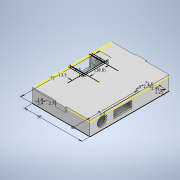
# Autodesk Inventor part: carcasaDisplayAdapter
Saved by Autodesk Inventor 2020 (Build 240168000, 168)
## iProperties
Created: 2021-04-22
Part Number: carcasaDisplayAdapter
Material: Generic
Document SubType Name: Modeling
Designer: Vlasciar
Density: 1 g/cm^3
Appearance: Default
Author: Vlasciar
Autodesk Inventor part; units mm, degrees
ref_plane "YZ Plane" through (0, 0, 0) normal (1, 0, 0) x (0, 1, 0)
ref_plane "XZ Plane" through (0, 0, 0) normal (0, 1, 0) x (-1, 0, 0)
ref_plane "XY Plane" through (0, 0, 0) normal (0, 0, 1) x (1, 0, 0)
sketch "Sketch1" plane through (0, 0, 0) normal (0, 1, 0) x (-1, 0, 0)
  line L0 (-28, -38.5) -> (28, -38.5)
  line L1 (28, -38.5) -> (28, 38.5)
  line L2 (28, 38.5) -> (-28, 38.5)
  line L3 (-28, 38.5) -> (-28, -38.5)
  line L4 (-28, -38.5) -> (28, 38.5) construction
  line L5 (28, -38.5) -> (-28, 38.5) construction
  point P0 (0, 0)
  dimension "d0" = 56
  dimension "d1" = 77
  constraints: 12 end point, 2 midpoint, 2 parallel, 1 horizontal, 1 perpendicular
  measures "d0" distance of L1.end L2.end
  measures "d1" distance of L0.end L1.end
extrude "Extrusion1" add sketch "Sketch1" along normal blind 12.5
shell "Shell1" thickness 1.5 removed faces 1 at (9.3333, 12.5, 12.8333)
sketch "Sketch2" plane through (28, 0, 38.5) normal (1, 0, 0) x (0, 0, -1)
  line L0 (0, 0) -> (77, 0) projected
  line L1 (0, 12.5) -> (77, 12.5) projected
  line L2 (14.3284, 3.5) -> (18, 3.5)
  circle A0 centre (11.5, 7) radius 4.5
  line L3 (1.5, 1.5) -> (1.5, 12.5) projected
  line L4 (40.75, 3.5) -> (23.25, 3.5)
  line L5 (23.25, 3.5) -> (23.25, 10.5)
  line L6 (23.25, 10.5) -> (40.75, 10.5)
  line L7 (40.75, 10.5) -> (40.75, 3.5)
  line L8 (40.75, 3.5) -> (23.25, 10.5) construction
  line L9 (23.25, 3.5) -> (40.75, 10.5) construction
  point P0 (38.5, 0)
  point P1 (32, 7)
  point P2 (32, 7)
  dimension "d10" = 9
  dimension "d7" = 3.5
  dimension "d8" = 3.5
  dimension "d9" = 5.5
  dimension "d11" = 5.5
  dimension "d12" = 17.5
  dimension "d13" = 7
  dimension "d14" = 21.75
  constraints: 14 end point, 3 midpoint, 2 horizontal, 2 parallel, 1 coincident, 1 horizontal alignment, 1 perpendicular, 3 other
  measures "d7" distance between parallel lines of L0 L2
  measures "d8" distance from line of L2 point (11.5, 7)
  measures "d9" distance from line of L1 point (11.5, 7)
  measures "d12" distance of L5.end L6.end
  measures "d13" distance of L6.end L4.start
  measures "d14" distance between parallel lines of L3 L5
extrude "Extrusion2" cut sketch "Sketch2" against normal blind 12.5
sketch "Sketch3" plane through (-28, 0, -38.5) normal (-1, 0, 0) x (0, 0, 1)
  line L0 (0, 0) -> (77, 0) projected
  line L1 (41.3, 3.5) -> (20.5, 3.5)
  line L2 (20.5, 3.5) -> (20.5, 6)
  line L3 (20.5, 6) -> (41.3, 6)
  line L4 (41.3, 6) -> (41.3, 3.5)
  line L5 (41.3, 3.5) -> (20.5, 6) construction
  line L6 (20.5, 3.5) -> (41.3, 6) construction
  line L7 (1.5, 1.5) -> (1.5, 12.5) projected
  line L8 (21.5, 6) -> (21.5, 3.5)
  line L9 (40.3, 6) -> (40.3, 3.4503)
  line L10 (0, 12.5) -> (77, 12.5) projected
  line L11 (21.5, 6) -> (21.5, 12.5)
  line L12 (1.5, 12.5) -> (75.5, 12.5) projected
  line L13 (40.3, 6) -> (40.3, 12.5)
  point P0 (38.5, 0)
  point P1 (30.9, 4.75)
  point P2 (40.3, 3.5)
  dimension "d17" = 3.5
  dimension "d18" = 2.5
  dimension "d19" = 20.8
  dimension "d20" = 19
  dimension "d21" = 1
  dimension "d22" = 1
  constraints: 20 end point, 4 point on line, 3 perpendicular, 2 midpoint, 2 parallel, 2 vertical, 1 horizontal
  measures "d17" distance between parallel lines of L0 L1
  measures "d18" distance of L3.end L1.start
  measures "d19" distance of L2.end L3.end
  measures "d20" distance between parallel lines of L7 L2
  measures "d21" distance between parallel lines of L8 L2
  measures "d22" distance between parallel lines of L4 L9
extrude "Extrusion3" cut sketch "Sketch3" against normal blind 12.5 contours L8 L3 L9 L1
sketch "Sketch4" plane through (-26.5, 1.5, -37) normal (0, 1, 0) x (1, 0, 0)
  line L0 (53, -74) -> (53, 0) projected
  line L1 (53, 0) -> (0, 0) projected
  line L2 (0, 0) -> (0, -74) projected
  line L3 (0, -74) -> (53, -74) projected
  circle A0 centre (3.175, -70.225) radius 1.375
  circle A1 centre (49.375, -3.825) radius 1.375
  point P0 (26.5, -37)
  dimension "d25" = 2.75
  dimension "d26" = 1.8
  dimension "d27" = 2.4
  dimension "d28" = 2.75
  dimension "d29" = 2.25
  dimension "d30" = 2.45
  constraints: 2 centre point
  measures "d25" diameter of A0
  measures "d26" distance edge to line of A0 L2
  measures "d27" distance edge to line of A0 L3
  measures "d28" diameter of A1
  measures "d29" distance edge to line of A1 L0
  measures "d30" distance edge to line of A1 L1
extrude "Extrusion4" add sketch "Sketch4" along normal blind 11 contours A0 | A1
extrude "Extrusion5" cut sketch "Sketch3" against normal blind 10 contours L11 L10 L13 L3
sketch "Sketch5" plane through (0, 12.5, 0) normal (0, 1, 0) x (1, 0, 0)
  line L0 (-28, -1.8) -> (-28, -38.5) projected
  line L1 (-28, -38.5) -> (28, -38.5) projected
  line L2 (28, -38.5) -> (28, 38.5) projected
  line L3 (28, 38.5) -> (-28, 38.5) projected
  line L4 (-28, 38.5) -> (-28, 17) projected
  line L5 (28, 38.5) -> (-28, 38.5) projected
  line L6 (28, 38.5) -> (-28, 38.5)
  line L7 (-28, 38.5) -> (-28, -38.5)
  line L8 (-28, -38.5) -> (28, -38.5)
  line L9 (28, -38.5) -> (28, 38.5)
  point P0 (0, 0)
  constraints: 8 end point, 2 parallel, 1 horizontal, 1 perpendicular
extrude "Extrusion6" add sketch "Sketch5" along normal blind 1.25 separate body
sketch "Sketch6" plane through (0, 13.75, 0) normal (0, 1, 0) x (1, 0, 0)
  line L0 (-28, 38.5) -> (-28, -38.5) projected
  line L1 (-26.5, -1.8) -> (-28, -1.8) projected
  line L2 (-28, -1.8) -> (0, -1.8)
  line L3 (-28, 17) -> (-28, -1.8) projected
  line L4 (-28, 17) -> (0, 17)
  line L5 (-14.5, 22) -> (-14.5, -18)
  line L6 (-14.5, -2.3) -> (-28, -2.3)
  line L7 (-28, 38.5) -> (-28, -38.5) projected
  line L8 (-14.5, 17.5) -> (-28, 17.5)
  line L9 (-14.5, -3.8) -> (-28, -3.8)
  line L10 (-14.5, 19) -> (-28, 19)
  line L11 (-14.5, 19) -> (-13, 19)
  line L12 (-13, 19) -> (-13, -3.8)
  line L13 (-13, -3.8) -> (-14.5, -3.8)
  line L14 (-14.5, -3.8) -> (-14.5, 19)
  line L15 (-26.5, 19) -> (-26.5, 17.5)
  line L16 (-26.5, 37) -> (-26.5, -37) projected
  line L17 (-26.5, -2.3) -> (-26.5, -3.8)
  point P0 (0, 0)
  point P1 (-26.5, -3.8)
  point P2 (-26.5, -2.3)
  dimension "d37" = 13.5
  dimension "d38" = 0.5
  dimension "d39" = 0.5
  dimension "d40" = 1.5
  dimension "d41" = 1.5
  dimension "d42" = 1.5
  dimension "d43" = 18.8
  constraints: 26 end point, 15 point on line, 6 perpendicular, 3 horizontal, 2 parallel, 1 horizontal alignment
  measures "d37" distance between parallel lines of L0 L5
  measures "d38" distance between parallel lines of L2 L6
  measures "d39" distance between parallel lines of L4 L8
  measures "d40" distance between parallel lines of L8 L10
  measures "d41" distance between parallel lines of L9 L6
  measures "d42" distance of L12.end L13.end
  measures "d43" distance between parallel lines of L2 L4
extrude "Extrusion7" cut sketch "Sketch6" against normal blind 1.25 contours L8 L16 L4 L0 | L4 L16 L1 L0 | L8 L5 L4 L16 | L1 L16 L6 L0 | L4 L5 L2 L16 | L2 L5 L6 L16 bodies 1
extrude "Extrusion9" add sketch "Sketch6" against normal blind 7 contours L10 L15 L8 L0 | L10 L5 L8 L15 | L11 L12 L4 L5 | L6 L16 L9 L0 | L4 L12 L2 L5 | L6 L5 L9 L16 | L2 L12 L13 L5 bodies 2
extrude "Extrusion10" cut sketch "Sketch6" against normal blind 7 contours L8 L16 L4 L0 | L4 L16 L1 L0 | L8 L5 L4 L16 | L1 L16 L6 L0 | L4 L5 L2 L16 | L2 L5 L6 L16 bodies 2
extrude "Extrusion11" cut sketch "Sketch6" against normal blind 7 contours L10 L15 L8 L0 | L6 L16 L9 L0 bodies 2
sketch "Sketch7" plane through (-26.5, 13.75, -19) normal (-1, 0, 0) x (0, 0, 1)
  line L0 (0, 0) -> (1.5, 0) projected
  line L1 (0, 0) -> (0, -1.25) projected
  line L2 (1.5, 0) -> (1.5, -7) projected
  line L3 (0, -1.25) -> (1.5, -1.25)
  line L4 (1.5, -1.25) -> (1.5, 0)
  line L5 (1.5, 0) -> (0, 0)
  line L6 (0, 0) -> (0, -1.25)
  line L7 (57.5, 0) -> (-19.5, 0) projected
  line L8 (-18, -1.25) -> (56, -1.25) projected
  line L9 (22.7673, 0) -> (21.3054, 0)
  line L10 (21.3054, 0) -> (21.3054, -1.25)
  line L11 (21.3054, -1.25) -> (22.7673, -1.25)
  line L12 (22.7673, -1.25) -> (22.7673, 0)
  point P0 (19, -13.75)
  constraints: 16 end point, 4 parallel, 2 horizontal, 2 perpendicular, 2 point on line
extrude "Extrusion12" add sketch "Sketch7" along normal blind 1.5 contours L0 L2 L3 L1 | L7 L12 L8 L10 bodies 2
sketch "Sketch8" plane through (-28, 0, 38.5) normal (0, 0, 1) x (1, 0, 0)
  line L0 (56, 0) -> (56, 12.5) projected
  line L1 (0, 12.5) -> (56, 12.5) projected
  line L2 (0, 0) -> (0, 12.5) projected
  line L3 (1.5, 12.5) -> (54.5, 12.5) projected
  line L4 (23, 12.5) -> (33, 12.5)
  line L5 (33, 12.5) -> (33, 9.5)
  line L6 (33, 9.5) -> (23, 9.5)
  line L7 (23, 9.5) -> (23, 12.5)
  point P0 (28, 0)
  point P1 (28, 12.5)
  dimension "d56" = 5
  dimension "d57" = 5
  dimension "d58" = 28
  dimension "d59" = 56
  dimension "d61" = 3
  constraints: 8 end point, 2 parallel, 1 horizontal, 1 midpoint, 1 perpendicular, 1 point on line
  measures "d56" distance from line of L7 point (28, 12.5)
  measures "d57" distance from line of L5 point (28, 12.5)
  measures "d58" distance from line of L0 point (28, 12.5)
  measures "d59" distance between parallel lines of L0 L2
  measures "d61" distance of L4.end L5.end
revolve "Revolution1" add sketch "Sketch8" angle 7 about axis through (-26.5, 12.5, 38.5) along (-1, 0, 0) bodies 1
mirror "Mirror1" about plane through (0, 0, 0) normal (0, 0, 1) of "Revolution1" bodies 1
sketch "Sketch9" plane through (-28, 12.5, 38.5) normal (0, 0, 1) x (1, 0, 0)
  line L0 (0, 0) -> (56, 0) projected
  line L1 (0, 1.25) -> (56, 1.25) projected
  line L2 (54.5, 0) -> (1.5, 0) projected
  line L3 (23, 0) -> (23, 1.25)
  line L4 (33, 0) -> (33, 1.25)
  point P0 (28, -12.5)
  point P1 (23, 0)
  constraints: 4 end point, 4 point on line, 1 parallel, 1 perpendicular
extrude "Extrusion13" add sketch "Sketch9" along normal blind 1 bodies 2
sketch "Sketch10" plane through (0, 12.5, 0) normal (0, -1, 0) x (1, 0, 0)
  line L0 (5, 38.5) -> (5, 39.5) projected
  line L1 (-5, 39.5) -> (5, 39.5) projected
  line L2 (-5, 38.5) -> (-5, 39.5) projected
  line L3 (5, 38.8656) -> (5, 38.5) projected
  line L4 (-5, 39.5) -> (5, 39.5)
  line L5 (5, 39.5) -> (5, 38.7485)
  line L6 (5, 38.7485) -> (-5, 38.7485)
  line L7 (-5, 38.7485) -> (-5, 39.5)
  point P0 (0, 0)
  constraints: 8 end point, 2 parallel, 1 horizontal, 1 perpendicular, 1 point on line
extrude "Extrusion14" add sketch "Sketch10" along normal blind 3 bodies 2
sketch "Sketch11" plane through (0, 9.5, 0) normal (0, -1, 0) x (1, 0, 0)
  line L0 (5, 39.5) -> (-5, 39.5) projected
  line L1 (-5, 39.5) -> (-5, 38.7485) projected
  line L2 (5, 38.7485) -> (5, 39.5) projected
  line L3 (5, 38.5) -> (5, 39.5) projected
  line L4 (-5, 39.5) -> (5, 39.5)
  line L5 (5, 39.5) -> (5, 39)
  line L6 (5, 39) -> (-5, 39)
  line L7 (-5, 39) -> (-5, 39.5)
  point P0 (0, 0)
  constraints: 8 end point, 2 parallel, 1 horizontal, 1 midpoint, 1 perpendicular
revolve "Revolution2" add sketch "Sketch11" angle 180 about axis through (5, 9.5, 39) along (1, 0, 0) bodies 2
sketch "Sketch12" plane through (-5, 9.5, 38.5) normal (-1, 0, 0) x (0, 0, 1)
  arc A0 (0, 0) -> (0.3656, 0.0224) centre (0, 3) ccw projected
  line L0 (0, 3) -> (0.3656, 0.0224) projected
  line L1 (0.2456, 1) -> (0.2456, 0)
  point P0 (-38.5, -9.5)
  point P1 (0.2456, 0.0101)
  constraints: 2 end point, 1 point on line, 1 vertical
extrude "Extrusion15" cut sketch "Sketch12" against normal blind 10 bodies 1
mirror "Mirror2" about plane through (0, 0, 0) normal (0, 0, 1) of "Extrusion13", "Extrusion14", "Revolution2" bodies 2
sketch "Sketch13" plane through (5, 9.5, -38.5) normal (1, 0, 0) x (0, 0, -1)
  arc A0 (0, 0) -> (0.3656, 0.0224) centre (0, 3) ccw projected
  line L0 (0.3656, 0.0224) -> (0, 3) projected
  line L1 (0, 3) -> (0.3656, 0.0224) projected
  line L2 (0.2456, 1) -> (0.2456, -0.0334)
  point P0 (-38.5, -9.5)
  point P1 (0.2456, 1)
  point P2 (0.2456, 0.0101)
  constraints: 2 end point, 1 point on line, 1 vertical
extrude "Extrusion16" cut sketch "Sketch13" against normal blind 10 bodies 1
sketch "Sketch14" plane through (0, 12.5, 0) normal (0, -1, 0) x (1, 0, 0)
  line L0 (28, 38.5) -> (28, -38.5) projected
  line L1 (26.5, -11.5) -> (25, -11.5)
  line L2 (25, -11.5) -> (25, -20.5)
  line L3 (25, -20.5) -> (26.5, -20.5)
  line L4 (26.5, -20.5) -> (26.5, -11.5)
  line L5 (5, 38.5) -> (28, 38.5) projected
  line L6 (26.5, 0) -> (18, 0)
  line L7 (26.5, 11.5) -> (25, 11.5)
  line L8 (25, 11.5) -> (25, 20.5)
  line L9 (25, 20.5) -> (26.5, 20.5)
  line L10 (26.5, 20.5) -> (26.5, 11.5)
  point P0 (0, 0)
  dimension "d71" = 9
  dimension "d72" = 1.5
  dimension "d73" = 1.5
  dimension "d76" = 50
  constraints: 18 end point, 4 symmetric about line, 2 horizontal, 2 parallel, 1 perpendicular, 1 vertical
  measures "d71" distance of L1.end L2.end
  measures "d72" distance between parallel lines of L0 L4
  measures "d73" distance of L2.end L3.end
  measures "d76" distance between parallel lines of L5 L1
extrude "Extrusion17" add sketch "Sketch14" along normal blind 2 contours L4 L3 L2 L1 bodies 2
extrude "Extrusion18" add sketch "Sketch14" along normal blind 2 contours L7 L8 L9 L10 bodies 2
body "Solid1"
body "Solid2"
